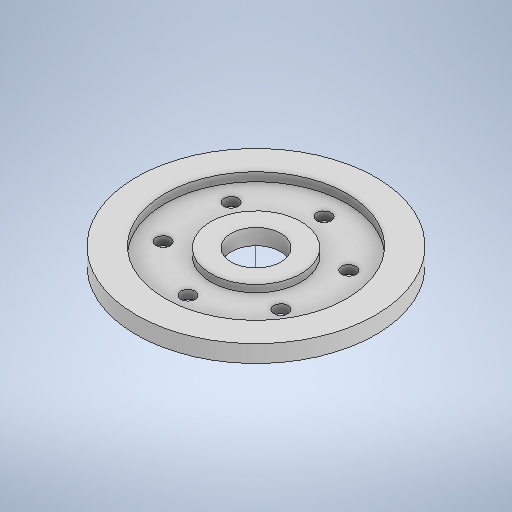
# Autodesk Inventor part: OuterBearingHolder
Saved by Autodesk Inventor 2027 (Build 310192060, 192F)
## iProperties
Created: 2026-07-06
Part Number: OuterBearingHolder
Material: Generic
Document SubType Name: Modeling
Designer: 13129
Density: 1 g/cm^3
Appearance: Default
Author: 13129
Autodesk Inventor part; units mm, degrees
ref_plane "YZ Plane" through (0, 0, 0) normal (1, 0, 0) x (0, 1, 0)
ref_plane "XZ Plane" through (0, 0, 0) normal (0, 1, 0) x (-1, 0, 0)
ref_plane "XY Plane" through (0, 0, 0) normal (0, 0, 1) x (1, 0, 0)
sketch "Sketch1" plane through (0, 0, 0) normal (0, 1, 0) x (-1, 0, 0)
  circle A0 centre (0, 0) radius 11
  circle A1 centre (0, 0) radius 20
  dimension "d0" = 22
  dimension "d1" = 40
  constraints: 2 centre point, 2 coincident
  measures "d0" diameter of A0
  measures "d1" diameter of A1
extrude "Extrusion1" add sketch "Sketch1" along normal blind 7
sketch "Sketch2" plane through (0, 0, 0) normal (1, 0, 0) x (0, 1, 0)
  line L0 (0, 40.32) -> (7.62, 40.32)
  line L1 (7.62, 40.32) -> (7.62, 53.02)
  line L2 (7.62, 53.02) -> (0, 53.02)
  line L3 (0, 53.02) -> (0, 40.32)
  line L4 (0, 40.32) -> (3.81, 40.32)
  line L5 (3.81, 40.32) -> (3.81, 20)
  line L6 (3.81, 20) -> (0, 20)
  line L7 (0, 20) -> (0, 40.32)
  line L8 (-1.524, 0) -> (9.144, 0) projected
  point P0 (0, 0)
  dimension "d4" = 20.32
  dimension "d5" = 7.62
  dimension "d6" = 20
  dimension "d7" = 3.81
  dimension "d8" = 12.7
  constraints: 16 end point, 4 parallel, 2 horizontal, 2 perpendicular, 1 vertical alignment
  measures "d4" distance of L4.end L5.end
  measures "d5" distance of L1.end L2.end
  measures "d6" distance from line of L6 point (0, 0)
  measures "d7" distance between parallel lines of L7 L5
  measures "d8" distance of L0.end L1.end
revolve "Revolution1" add sketch "Sketch2" angle 360 about axis through (0, -10, 0) along (0, 1, 0)
sketch "Sketch3" plane through (0, 3.81, 0) normal (0, 1, 0) x (1, 0, 0)
  circle A0 centre (0, 0) radius 40.32 construction
  circle A1 centre (0, 0) radius 20 construction
  circle A2 centre (0, 30.16) radius 3.175
  line L0 (0, 30.16) -> (0, 20)
  line L1 (0, 30.16) -> (0, 40.32)
  circle A3 centre (-26.1193, 15.08) radius 3.175
  circle A4 centre (-26.1193, -15.08) radius 3.175
  circle A5 centre (0, -30.16) radius 3.175
  circle A6 centre (26.1193, -15.08) radius 3.175
  circle A7 centre (26.1193, 15.08) radius 3.175
  dimension "d10" = 6.35
  dimension "d13" = 360
  constraints: 6 centre point, 4 end point, 3 vertical alignment, 2 vertical, 1 collinear, 15 other
  measures "d10" diameter of A2
extrude "Extrusion2" cut sketch "Sketch3" against normal blind 7
body "Solid1"
